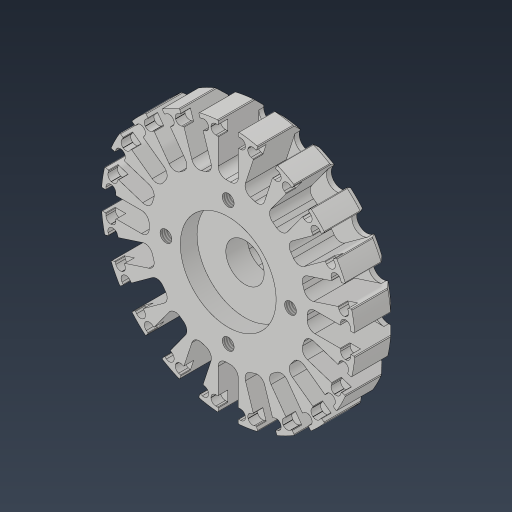
# Autodesk Inventor part: Radkasten
Saved by Autodesk Inventor 2023.1 (Build 271208000, 208)
## iProperties
Part Number: Radkasten
Material: Generisch
Document SubType Name: Modeling
Designer: rYan
Density: 1 g/cm^3
Appearance: Vorgabe
Mass: 11.5434 g
Surface Area: 96.0365 cm^2
Volume: 11.5434 cm^3
Author: rYan
Autodesk Inventor part; units mm, degrees
ref_plane "YZ Plane" through (0, 0, 0) normal (1, 0, 0) x (0, 1, 0)
ref_plane "XZ Plane" through (0, 0, 0) normal (0, 1, 0) x (-1, 0, 0)
ref_plane "XY Plane" through (0, 0, 0) normal (0, 0, 1) x (1, 0, 0)
sketch "Skizze1" plane through (0, 0, 0) normal (0, 0, 1) x (1, 0, 0)
  line L0 (0, 0) -> (0, 10)
  line L1 (4, 0) -> (4, 10)
  line L2 (4, 10) -> (5.8, 10)
  line L3 (5.8, 10) -> (5.8, 8.8)
  line L4 (21, 9.5) -> (26.5, 9.5)
  line L5 (26.5, 9.5) -> (26.5, 0)
  line L6 (26.5, 0) -> (4, 0)
  line L7 (-5.3, 0) -> (31.8, 0) projected
  line L8 (15.9, 10) -> (15.9, 8.8)
  line L9 (15.9, 8.8) -> (5.8, 8.8)
  line L10 (21, 9.5) -> (21, 9.5)
  line L11 (15.9, 10) -> (15.9, 11.6)
  line L12 (15.9, 11.6) -> (17.1, 11.6)
  line L13 (17.1, 11.6) -> (17.1, 9.5)
  line L14 (15.9, 10) -> (15.9, 10)
  line L15 (17.1, 9.5) -> (21, 9.5)
  line L16 (16.5, 11.6) -> (16.5, 0) construction
  dimension "d0" = 8
  dimension "d1" = 53
  dimension "d2" = 9.5
  dimension "d4" = 11.6
  dimension "d24" = 1.2
  dimension "d34" = 10
  dimension "d35" = 42
  dimension "d71" = 33
  dimension "d72" = 1.2
  dimension "d80" = 11.6
  constraints: 32 end point, 9 perpendicular, 5 point on line, 4 vertical, 3 horizontal, 1 collinear, 1 midpoint, 1 parallel
  measures "d0" diameter of L1 L0
  measures "d1" diameter of L5 L0
  measures "d2" distance of L4.end L5.end
  measures "d4" diameter of L3 L0
  measures "d24" distance of L8.start L8.end
  measures "d34" distance of L1.start L1.end
  measures "d35" diameter of L10 L0
  measures "d71" diameter of L16 L0
  measures "d72" distance of L11.end L12.end
  measures "d80" distance between parallel lines of L6 L12
revolve "Umdrehung1" add sketch "Skizze1" angle 360 about axis through (0, 0, 0) along (0, 1, 0)
sketch "Skizze2" plane through (0, 0, 0) normal (0, 1, 0) x (-1, 0, 0)
  circle A0 centre (0, 0) radius 26.5 projected
  circle A1 centre (0, 0) radius 16.5 construction
  line L0 (2.1, 26.5) -> (-2.1, 26.5)
  line L1 (-2.1, 26.5) -> (-2.1, 18.1)
  line L2 (-0.5, 16.5) -> (0.5, 16.5)
  line L3 (2.1, 18.1) -> (2.1, 26.5)
  line L4 (0, 0) -> (0, 26.5) construction
  arc A2 (0.5, 16.5) -> (2.1, 18.1) centre (0.5, 18.1) ccw
  arc A3 (-2.1, 18.1) -> (-0.5, 16.5) centre (-0.5, 18.1) ccw
  dimension "d6" = 1.6
  dimension "d7" = 4.2
  dimension "d8" = 33
  constraints: 10 end point, 5 tangent, 4 point on circle, 3 centre point, 2 parallel, 1 coincident, 1 equal radius, 1 horizontal, 1 midpoint, 1 perpendicular, 1 vertical, 1 vertical alignment, 2 other
  measures "d6" radius of A2
  measures "d7" distance between parallel lines of L1 L3
  measures "d8" diameter of A1
extrude "Querrolle" cut sketch "Skizze2" along normal blind 8.5 contours L3 A2 L2 A3 L1 A0 | A0 L0 L3 | L1 L0 A0 picked at (0, 20.9)
fillet "Rundung2" radius 0.15 2 edges at (2.1, 4.25, 26.4167) (-2.1, 4.25, 26.4167)
sketch "Skizze10" plane through (0, 8.5, 0) normal (0, -1, 0) x (1, 0, 0)
  line L0 (-2.1, 18.1) -> (-2.1, 26.2538) projected
  line L1 (-2.1, 18.1) -> (-2.1, 26.2538) projected
  line L2 (2.1, 26.2538) -> (2.1, 18.1) projected
  line L3 (2.1, 26.2538) -> (2.1, 18.1) projected
  circle A0 centre (0, 0) radius 26.5 projected
  arc A1 (-2.1, 24) -> (2.1, 24) centre (0, 24) ccw
  line L4 (2.1, 24) -> (2.1, 26.5)
  line L5 (2.1, 26.5) -> (-2.1, 26.5)
  line L6 (-2.1, 26.5) -> (-2.1, 24)
  point P0 (-2.1, 26.4167)
  point P1 (-2.1, 26.4167)
  point P2 (2.1, 26.4167)
  point P3 (2.1, 26.4167)
  dimension "d77" = 2.5
  constraints: 6 end point, 3 point on line, 3 tangent, 2 point on circle, 1 centre point, 1 horizontal, 1 parallel
  measures "d77" distance from line of L5 A1.centre
extrude "Durchbruch" cut sketch "Skizze10" against normal through all contours L0 L6 A0 L4 L2 A1 | L6 L5 A0 | L5 L4 A0 picked at (0, 24.8333)
sketch "Skizze3" plane through (0, 0, 0) normal (0, 1, 0) x (-1, 0, 0)
  line L0 (2.6, 25.525) -> (-2.6, 25.525)
  line L1 (-3.6, 24.525) -> (-3.6, 24.475)
  line L2 (-2.6, 23.475) -> (2.6, 23.475)
  line L3 (3.6, 24.475) -> (3.6, 24.525)
  line L4 (0, -5.1464) -> (0, 30.8785) projected
  line L5 (2.65, 25.504) -> (-2.65, 25.504) construction
  line L6 (-2.65, 25.504) -> (-2.65, 23.496) construction
  line L7 (-2.65, 23.496) -> (2.65, 23.496) construction
  line L8 (2.65, 23.496) -> (2.65, 25.504) construction
  line L9 (-2.65, 25.504) -> (-3, 25.4102) construction
  line L10 (-3, 25.4102) -> (-3, 23.5898) construction
  line L11 (-3, 23.5898) -> (-2.65, 23.496) construction
  line L12 (2.65, 25.504) -> (3, 25.4102) construction
  line L13 (3, 25.4102) -> (3, 23.5898) construction
  line L14 (3, 23.5898) -> (2.65, 23.496) construction
  line L15 (3, 24.5) -> (-3, 24.5) construction
  line L16 (0, 25.504) -> (0, 23.496) construction
  arc A0 (3.6, 24.525) -> (2.6, 25.525) centre (2.6, 24.525) ccw
  arc A1 (-2.6, 25.525) -> (-3.6, 24.525) centre (-2.6, 24.525) ccw
  arc A2 (-3.6, 24.475) -> (-2.6, 23.475) centre (-2.6, 24.475) ccw
  arc A3 (2.6, 23.475) -> (3.6, 24.475) centre (2.6, 24.475) ccw
  line L17 (3.6, 24.5) -> (-3.6, 24.5) construction
  line L18 (2.1, 18.1) -> (2.1, 26.2538) projected
  line L19 (3.375, 24.75) -> (2.6, 25.525) construction
  line L20 (2.6, 25.525) -> (-2.6, 25.525) construction
  line L21 (-2.6, 25.525) -> (-3.375, 24.75) construction
  line L22 (-3.375, 24.75) -> (-3.375, 24.5) construction
  line L23 (3.375, 24.75) -> (3.375, 24.5) construction
  point P0 (0, 0)
  point P1 (3.6, 25.525)
  point P2 (-3.6, 25.525)
  point P3 (2.65, 24.5)
  point P4 (-2.65, 24.5)
  point P5 (0, 24.5)
  point P6 (0, 24.5)
  dimension "d11" = 2.05
  dimension "d12" = 7.2
  dimension "d13" = 2.008
  dimension "d14" = 15
  dimension "d15" = 0.35
  dimension "d16" = 6
  dimension "d17" = 1
  dimension "d18" = 24.5
  dimension "d82" = 0.55
  dimension "d83" = 0.5
  dimension "d84" = 45
  dimension "d85" = 1.025
  dimension "d86" = 0.5
  dimension "d87" = 0.25
  constraints: 44 end point, 11 midpoint, 9 point on line, 8 point on circle, 8 tangent, 5 parallel, 4 centre point, 4 perpendicular, 3 equal radius, 3 horizontal, 1 vertical, 6 other
  measures "d11" distance between parallel lines of L0 L2
  measures "d12" distance of point (3.6, 25.525) point (-3.6, 25.525)
  measures "d13" distance between parallel lines of L7 L5
  measures "d14" angle of L5 L9
  measures "d15" distance between parallel lines of L6 L10
  measures "d16" distance between parallel lines of L10 L13
  measures "d17" radius of A0
  measures "d18" distance from line of L17 point (0, 0)
  measures "d82" distance from line of L5.start L18
  measures "d83" distance from line of L0.start L18
  measures "d84" angle of L20 L21
  measures "d85" distance between parallel lines of L15 L20
  measures "d86" distance from line of L18 L19.end
  measures "d87" distance from line of L17 L19.start
extrude "Achse" cut sketch "Skizze3" along normal blind 2
fillet "Rundung1" radius 0.1 4 edges at (-2.1, 1, 25.525) (-2.1, 1, 23.475) (2.1, 1, 25.525) (2.1, 1, 23.475)
pattern_circular "Runde Anordnung1" count 20 over 360 about axis through (0, -10, 0) along (0, 1, 0) of "Querrolle", "Achse", "Rundung1", "Durchbruch", "Rundung2"
sketch "Skizze4" plane through (0, 0, 0) normal (0, 1, 0) x (-1, 0, 0)
  circle A0 centre (0, 0) radius 13 construction
  line L0 (13, 0) -> (-13, 0) construction
  line L1 (0, 13) -> (0, -13) construction
  line L2 (0, -18.2) -> (0, 18.2) projected
  line L3 (-18.2, 0) -> (18.2, 0) projected
  dimension "d26" = 26
  constraints: 5 coincident, 4 end point, 4 point on circle, 2 collinear, 1 centre point, 1 horizontal, 1 perpendicular
  measures "d26" diameter of A0
hole "Bohrung1" at (0, 0, -13) at (0, 0, 13) at (-13, 0, 0) at (13, 0, 0) direction (0, 1, 0) diameter 2.459 depth 7 tip angle 118 thread size "M3x0.5" class "6H" standard "ISO Metric profile"
sketch "Skizze6" plane through (0.25, 8.8, 18) normal (0, -1, 0) x (0.7071068, 0, -0.7071068)
  circle A0 centre (12.5511, -12.9047) radius 8.5 construction
  line L0 (4.0511, -12.9047) -> (21.0511, -12.9047) construction
  line L1 (12.5511, -21.4047) -> (12.5511, -4.4047) construction
  dimension "d48" = 17
  constraints: 5 coincident, 4 end point, 4 midpoint, 4 point on circle, 1 centre point, 1 horizontal, 1 perpendicular
  measures "d48" diameter of A0
hole "Fräshilfe" [suppressed]
chamfer "Fase1" distance 2 angle 45 20 edges at (4.1455, 9.5, 26.1737) (12.0307, 9.5, 23.6117) (18.7383, 9.5, 18.7383) (23.6117, 9.5, 12.0307) (26.1737, 9.5, 4.1455) (26.1737, 9.5, -4.1455) (23.6117, 9.5, -12.0307) (18.7383, 9.5, -18.7383) (12.0307, 9.5, -23.6117) (4.1455, 9.5, -26.1737) (-4.1455, 9.5, -26.1737) (-12.0307, 9.5, -23.6117) (-18.7383, 9.5, -18.7383) (-23.6117, 9.5, -12.0307) (-26.1737, 9.5, -4.1455) (-26.1737, 9.5, 4.1455) (-23.6117, 9.5, 12.0307) (-18.7383, 9.5, 18.7383) (-12.0307, 9.5, 23.6117) (-4.1455, 9.5, 26.1737)
sketch "Skizze7" plane through (0, 10, 0) normal (0, 1, 0) x (1, 0, 0)
  circle A0 centre (0, 0) radius 5.8 projected
  circle A1 centre (0, 0) radius 5.1113 construction
  circle A2 centre (0, 0) radius 4 projected
  line L0 (2.2, 4.2) -> (-2.2, 4.2)
  line L1 (-4.2, 2.2) -> (-4.2, -2.2)
  line L2 (-2.2, -4.2) -> (2.2, -4.2)
  line L3 (4.2, -2.2) -> (4.2, 2.2)
  arc A3 (4.2, 2.2) -> (2.2, 4.2) centre (2.2, 2.2) ccw
  arc A4 (2.2, -4.2) -> (4.2, -2.2) centre (2.2, -2.2) ccw
  arc A5 (-4.2, -2.2) -> (-2.2, -4.2) centre (-2.2, -2.2) ccw
  arc A6 (-2.2, 4.2) -> (-4.2, 2.2) centre (-2.2, 2.2) ccw
  line L4 (2.2, 2.2) -> (-2.2, -2.2) construction
  line L5 (2.2, -2.2) -> (-2.2, 2.2) construction
  line L6 (0, 37.1) -> (0, -37.1) projected
  line L7 (37.1, 0) -> (-37.1, 0) projected
  dimension "d60" = 2
  dimension "d66" = 8.4
  constraints: 12 end point, 9 tangent, 8 point on circle, 5 centre point, 3 equal radius, 2 midpoint, 2 parallel, 2 perpendicular, 1 coincident, 1 horizontal, 2 other
  measures "d60" radius of A3
  measures "d66" distance between parallel lines of L0 L2
extrude "Extrusion3" cut sketch "Skizze7" against normal blind 2 contours L7 A2 L6 L0 A3 L3 | L3 A4 L2 L6 A2 L7 | L6 A2 L7 L1 A6 L0 | L2 A5 L1 L7 A2 L6
sketch "Skizze8" plane through (0.5, 0, 18.1) normal (0, -1, 0) x (0.7071068, 0, -0.7071068)
  circle A0 centre (12.4451, -13.1522) radius 4 projected
  circle A1 centre (12.4451, -13.1522) radius 10
  dimension "d63" = 20
  constraints: 1 centre point, 1 coincident
  measures "d63" diameter of A1
extrude "Extrusion4" cut sketch "Skizze8" against normal blind 3.5
